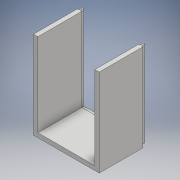
# Autodesk Inventor part: tb3_start_walls_v2
Saved by Autodesk Inventor 2017 (Build 210142000, 142)
## iProperties
Created: 2017-04-11
Part Number: tb3_start_walls_v2
Material: Generic
Document SubType Name: Modeling
Designer: PC
Density: 1 g/cm^3
Appearance: Default
Author: PC
Autodesk Inventor part; units mm, degrees
ref_plane "YZ Plane" through (0, 0, 0) normal (1, 0, 0) x (0, 1, 0)
ref_plane "XZ Plane" through (0, 0, 0) normal (0, 1, 0) x (-1, 0, 0)
ref_plane "XY Plane" through (0, 0, 0) normal (0, 0, 1) x (1, 0, 0)
sketch "Sketch1" plane through (0, 0, 0) normal (0, 1, 0) x (-1, 0, 0)
  line L0 (-37.5, -50) -> (37.5, -50)
  line L1 (37.5, -50) -> (37.5, 50)
  line L2 (37.5, 50) -> (-37.5, 50)
  line L3 (-37.5, 50) -> (-37.5, -50)
  line L4 (-37.5, -50) -> (37.5, 50) construction
  line L5 (37.5, -50) -> (-37.5, 50) construction
  point P0 (0, 0)
  dimension "d0" = 75
  dimension "d1" = 100
  constraints: 12 end point, 2 midpoint, 2 parallel, 1 horizontal, 1 perpendicular
  measures "d0" distance of L2.end L1.end
  measures "d1" distance of L1.end L0.end
extrude "Extrusion1" add sketch "Sketch1" along normal blind 50
sketch "Sketch2" plane through (0, 50, 0) normal (0, 1, 0) x (1, 0, 0)
  line L0 (-37.5, -50) -> (37.5, -50) projected
  line L1 (-32.5, -50) -> (32.5, -50)
  line L2 (32.5, -50) -> (32.5, 45)
  line L3 (32.5, 45) -> (-32.5, 45)
  line L4 (-32.5, 45) -> (-32.5, -50)
  point P0 (0, 0)
  dimension "d4" = 65
  dimension "d5" = 95
  constraints: 8 end point, 2 parallel, 1 horizontal, 1 perpendicular, 1 point on line
  measures "d4" distance of L3.end L2.end
  measures "d5" distance of L2.end L1.end
extrude "Extrusion2" cut sketch "Sketch2" against normal blind 50
sketch "Sketch3" plane through (0, 50, 0) normal (0, 1, 0) x (1, 0, 0)
  line L0 (-37.5, -50) -> (-32.5, -50) projected
  line L1 (-36, -50) -> (-34, -50)
  line L2 (-34, -50) -> (-34, 48.5)
  line L3 (-34, 48.5) -> (-36, 48.5)
  line L4 (-36, 48.5) -> (-36, -50)
  line L5 (-36, 48.5) -> (36, 48.5)
  line L6 (36, 48.5) -> (36, 46.5)
  line L7 (36, 46.5) -> (-36, 46.5)
  line L8 (-36, 46.5) -> (-36, 48.5)
  line L9 (36, 48.5) -> (34, 48.5)
  line L10 (34, 48.5) -> (34, -50)
  line L11 (34, -50) -> (36, -50)
  line L12 (36, -50) -> (36, 48.5)
  point P0 (0, 0)
  dimension "d8" = 2
  dimension "d9" = 98.5
  dimension "d10" = 72
  dimension "d11" = 2
  constraints: 24 end point, 6 parallel, 3 horizontal, 3 perpendicular, 2 point on line
  measures "d8" distance of L3.end L2.end
  measures "d9" distance of L2.end L1.end
  measures "d10" distance of L6.end L7.end
  measures "d11" distance of L5.end L6.end
extrude "Extrusion3" add sketch "Sketch3" along normal blind 4
sketch "Sketch4" plane through (36, 50, 50) normal (1, 0, 0) x (0, 0, -1)
  line L0 (0, 0) -> (100, 0) projected
  line L1 (98.5, 0) -> (98.5, 4) projected
  line L2 (0, 0) -> (98.5, 0)
  line L3 (98.5, 0) -> (98.5, 4)
  line L4 (98.5, 4) -> (0, 4)
  line L5 (0, 4) -> (0, 0)
  point P0 (50, -50)
  constraints: 8 end point, 2 parallel, 1 horizontal, 1 perpendicular
extrude "Extrusion4" cut sketch "Sketch4" against normal blind 0.25
sketch "Sketch5" plane through (34, 50, -46.5) normal (-1, 0, 0) x (0, 0, 1)
  line L0 (96.5, 0) -> (96.5, 4) projected
  line L1 (96.5, 0) -> (0, 0) projected
  line L2 (96.5, 4) -> (0, 4)
  line L3 (0, 4) -> (0, 0)
  line L4 (0, 0) -> (96.5, 0)
  line L5 (96.5, 0) -> (96.5, 4)
  point P0 (46.5, -50)
  constraints: 8 end point, 2 parallel, 1 horizontal, 1 perpendicular
extrude "Extrusion5" cut sketch "Sketch5" against normal blind 0.25
sketch "Sketch6" plane through (-36, 50, -48.5) normal (0, 0, -1) x (-1, 0, 0)
  line L0 (-71.75, 4) -> (0, 4) projected
  line L1 (0, 0) -> (-71.75, 0) projected
  line L2 (0, 4) -> (-71.75, 4)
  line L3 (-71.75, 4) -> (-71.75, 0)
  line L4 (-71.75, 0) -> (0, 0)
  line L5 (0, 0) -> (0, 4)
  point P0 (-36, -50)
  constraints: 8 end point, 2 parallel, 1 horizontal, 1 perpendicular
extrude "Extrusion6" cut sketch "Sketch6" against normal blind 0.25
sketch "Sketch7" plane through (-34, 50, 50) normal (1, 0, 0) x (0, 0, -1)
  line L0 (0, 0) -> (0, 4) projected
  line L1 (0, 4) -> (96.5, 4) projected
  line L2 (0, 0) -> (96.5, 0)
  line L3 (96.5, 0) -> (96.5, 4)
  line L4 (96.5, 4) -> (0, 4)
  line L5 (0, 4) -> (0, 0)
  point P0 (50, -50)
  constraints: 8 end point, 2 parallel, 1 horizontal, 1 perpendicular
extrude "Extrusion7" cut sketch "Sketch7" against normal blind 0.25
sketch "Sketch8" plane through (-36, 50, 50) normal (-1, 0, 0) x (0, 0, 1)
  line L0 (0, 4) -> (-96.5, 4) projected
  line L1 (-98.25, 0) -> (0, 0) projected
  line L2 (0, 4) -> (-98.25, 4)
  line L3 (-98.25, 4) -> (-98.25, 0)
  line L4 (-98.25, 0) -> (0, 0)
  line L5 (0, 0) -> (0, 4)
  point P0 (-50, -50)
  constraints: 8 end point, 2 parallel, 1 horizontal, 1 perpendicular
extrude "Extrusion8" cut sketch "Sketch8" against normal blind 0.25
sketch "Sketch9" plane through (-36, 50, -48.25) normal (0, 0, -1) x (-1, 0, 0)
  line L0 (-72, 4) -> (0, 4)
  line L1 (0, 4) -> (0, 0)
  line L2 (0, 0) -> (-72, 0)
  line L3 (-72, 0) -> (-72, 4)
  point P0 (-36, -50)
  constraints: 8 end point, 2 parallel, 1 horizontal, 1 perpendicular
extrude "Extrusion9" cut sketch "Sketch9" against normal blind 0.25
body "Solid1"
